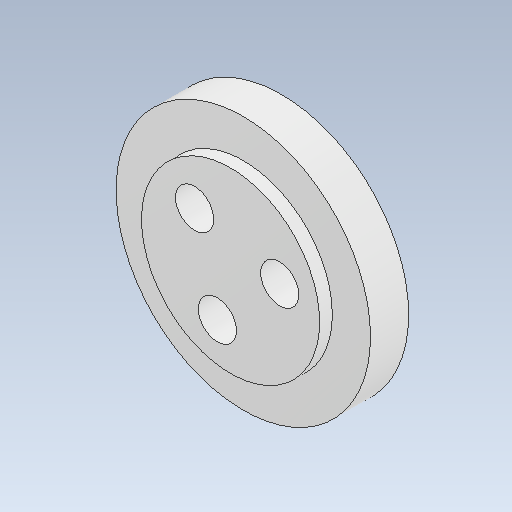
# Autodesk Inventor part: カムD14
Saved by Autodesk Inventor 2020.2 (Build 242310000, 310)
## iProperties
Created: 2020-03-20
Part Number: カムD14
Material: アセタール樹脂、白
Document SubType Name: Modeling
Designer: aoyam
Density: 1.425 g/cm^3
Appearance: 滑らか - 白
Mass: 1.44152 g
Surface Area: 9.31482 cm^2
Volume: 1.01159 cm^3
Author: aoyam
Autodesk Inventor part; units mm, degrees
ref_plane "YZ Plane" through (0, 0, 0) normal (1, 0, 0) x (0, 1, 0)
ref_plane "XZ Plane" through (0, 0, 0) normal (0, 1, 0) x (-1, 0, 0)
ref_plane "XY Plane" through (0, 0, 0) normal (0, 0, 1) x (1, 0, 0)
sketch "スケッチ1" plane through (0, 0, 0) normal (0, 0, 1) x (1, 0, 0)
  circle A0 centre (0, 0) radius 7
  circle A1 centre (-2.8284, 2.8284) radius 1.5
  circle A2 centre (-1.0353, -3.8637) radius 1.5
  circle A3 centre (3.8637, 1.0353) radius 1.5
  circle A4 centre (0, 0) radius 10
  dimension "d0" = 14
  dimension "d1" = 3
  dimension "d2" = 4
  dimension "d5" = 360
  dimension "d9" = 20
  constraints: 5 centre point, 2 coincident, 7 other
  measures "d0" diameter of A0
  measures "d1" diameter of A1
  measures "d2" distance of A1.centre point (0, 0)
  measures "d9" diameter of A4
extrude "押し出し1" add sketch "スケッチ1" along normal blind 4 contours A0
extrude "押し出し2" add sketch "スケッチ1" along normal blind 3 contours A4
